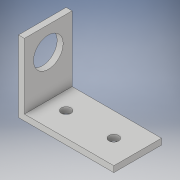
# Autodesk Inventor part: Piston bracket
Saved by Autodesk Inventor 2018 (Build 220112000, 112)
## iProperties
Created: 2019-01-25
Part Number: Piston bracket
Material: Generic
Document SubType Name: Modeling
Designer: s-2512711
Density: 1 g/cm^3
Appearance: Default
Author: s-2512711
Autodesk Inventor part; units mm, degrees
ref_plane "YZ Plane" through (0, 0, 0) normal (1, 0, 0) x (0, 1, 0)
ref_plane "XZ Plane" through (0, 0, 0) normal (0, 1, 0) x (-1, 0, 0)
ref_plane "XY Plane" through (0, 0, 0) normal (0, 0, 1) x (1, 0, 0)
sketch "Sketch1" plane through (0, 0, 0) normal (0, 0, 1) x (1, 0, 0)
  line L0 (0, 0) -> (3.175, 0)
  line L1 (3.175, 0) -> (3.175, 38.1)
  line L2 (3.175, 38.1) -> (0, 38.1)
  line L3 (0, 38.1) -> (0, 0)
  line L4 (0, 0) -> (50.8, 0)
  line L5 (50.8, 0) -> (50.8, 3.175)
  line L6 (50.8, 3.175) -> (0, 3.175)
  line L7 (0, 3.175) -> (0, 0)
  dimension "d0" = 3.175
  dimension "d1" = 38.1
  dimension "d2" = 50.8
  dimension "d3" = 3.175
  constraints: 16 end point, 4 parallel, 2 horizontal, 2 perpendicular
  measures "d0" distance of L2.end L1.end
  measures "d1" distance of L1.end L0.end
  measures "d2" distance of L6.end L5.end
  measures "d3" distance of L5.end L4.end
extrude "Extrusion1" add sketch "Sketch1" along normal blind 25.4
sketch "Sketch2" plane through (3.175, 3.175, 0) normal (1, 0, 0) x (0, 0, -1)
  line L0 (0, 34.925) -> (-25.4, 34.925) projected
  line L1 (-12.7, 34.925) -> (-12.7, 9.525)
  circle A0 centre (-12.7, 22.225) radius 7.9057
  point P0 (0, -3.175)
  dimension "d6" = 25.4
  dimension "d7" = 15.8115
  constraints: 2 end point, 2 midpoint, 1 centre point, 1 vertical
  measures "d6" distance of L1.start L1.end
  measures "d7" diameter of A0
extrude "Extrusion2" cut sketch "Sketch2" against normal blind 25.4
sketch "Sketch3" plane through (3.175, 3.175, 0) normal (0, 1, 0) x (1, 0, 0)
  line L0 (47.625, 0) -> (47.625, -25.4) construction
  line L1 (47.625, -12.7) -> (34.925, -12.7) construction
  line L2 (47.625, -12.7) -> (60.325, -12.7) construction
  circle A0 centre (34.925, -12.7) radius 2.5797
  line L3 (34.925, -12.7) -> (9.525, -12.7) construction
  circle A1 centre (9.525, -12.7) radius 2.5797
  point P0 (-3.175, 0)
  dimension "d10" = 12.7
  dimension "d11" = 180
  dimension "d12" = 5.1594
  dimension "d15" = 25.4
  constraints: 6 end point, 3 horizontal, 2 centre point, 2 coincident, 1 collinear, 1 midpoint
  measures "d10" distance of L1.start L1.end
  measures "d11" angle of L1 L2
  measures "d12" diameter of A0
  measures "d15" distance of L3.start L3.end
extrude "Extrusion4" cut sketch "Sketch3" against normal blind 25.4
body "Solid1"
